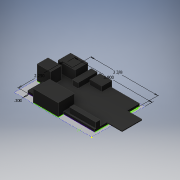
# Autodesk Inventor part: comp
Saved by Autodesk Inventor 2018 (Build 220112000, 112)
## iProperties
Created: 2018-03-12
Part Number: comp
Material: Generic
Document SubType Name: Modeling
Designer: Josh
Density: 1 g/cm^3
Appearance: Glossy - Black
Author: Josh
Autodesk Inventor part; units mm, degrees
ref_plane "YZ Plane" through (0, 0, 0) normal (1, 0, 0) x (0, 1, 0)
ref_plane "XZ Plane" through (0, 0, 0) normal (0, 1, 0) x (-1, 0, 0)
ref_plane "XY Plane" through (0, 0, 0) normal (0, 0, 1) x (1, 0, 0)
sketch "Sketch1" plane through (0, 0, 0) normal (0, 1, 0) x (-1, 0, 0)
  line L0 (0, 0) -> (99.06, 0) construction
  line L1 (99.06, 0) -> (99.06, -67.803) construction
  line L2 (99.06, -67.803) -> (0, -67.803) construction
  line L3 (0, -67.803) -> (0, 0) construction
  line L4 (3.6636, -7.62) -> (89.3886, -7.62)
  line L5 (89.3886, -7.62) -> (89.3886, -64.77)
  line L6 (89.3886, -64.77) -> (3.6636, -64.77)
  line L7 (3.6636, -64.77) -> (3.6636, -7.62)
  line L8 (79.4904, -27.0781) -> (96.8098, -27.0781)
  line L9 (96.8098, -27.0781) -> (96.8098, -40.9573)
  line L10 (96.8098, -40.9573) -> (79.4904, -40.9573)
  line L11 (79.4904, -40.9573) -> (79.4904, -27.0781)
  line L12 (90.7598, -47.719) -> (68.9327, -47.719)
  line L13 (68.9327, -47.719) -> (68.9327, -63.8522)
  line L14 (68.9327, -63.8522) -> (90.7598, -63.8522)
  line L15 (90.7598, -63.8522) -> (90.7598, -47.719)
  line L16 (55.7859, -66.2925) -> (40.4182, -66.2925)
  line L17 (40.4182, -66.2925) -> (40.4182, -53.4684)
  line L18 (40.4182, -53.4684) -> (55.7859, -53.4684)
  line L19 (55.7859, -53.4684) -> (55.7859, -66.2925)
  line L20 (9.1527, -52.5145) -> (2.1577, -52.5145)
  line L21 (2.1577, -52.5145) -> (2.1577, -61.4172)
  line L22 (2.1577, -61.4172) -> (9.1527, -61.4172)
  line L23 (9.1527, -61.4172) -> (9.1527, -52.5145)
  line L24 (37.3446, -14.572) -> (3.6636, -14.572)
  line L25 (3.6636, -14.572) -> (3.6636, -9.0608)
  line L26 (3.6636, -9.0608) -> (37.3446, -9.0608)
  line L27 (37.3446, -9.0608) -> (37.3446, -14.572)
  line L28 (43.4917, -21.567) -> (75.2871, -21.567)
  line L29 (75.2871, -21.567) -> (75.2871, -0.688)
  line L30 (75.2871, -0.688) -> (43.4917, -0.688)
  line L31 (43.4917, -0.688) -> (43.4917, -21.567)
  line L32 (66.6334, -41.9689) -> (59.3894, -41.9689)
  line L33 (59.3894, -41.9689) -> (59.3894, -66.2925)
  line L34 (59.3894, -66.2925) -> (66.6334, -66.2925)
  line L35 (66.6334, -66.2925) -> (66.6334, -41.9689)
  point P0 (15.875, 0)
  dimension "d6" = 99.06
  dimension "d18" = 85.725
  dimension "d19" = 57.15
  dimension "d20" = 7.62
  constraints: 64 end point, 16 parallel, 8 horizontal, 8 perpendicular, 2 point on line, 2 other
  measures "d6" distance of L1.end L2.end
  measures "d18" distance of L5.end L6.end
  measures "d19" distance of L4.end L5.end
  measures "d20" distance between parallel lines of L0 L4
extrude "Extrusion1" add sketch "Sketch1" along normal blind 3.175 contours L4 L31 L28 L29 L5 L8 L11 L10 L12 L13 L14 L6 L35 L32 L33 L19 L18 L17 L7 L22 L23 L20 L24 L27 L26 | L4 L29 L28 L31 | L26 L27 L24 L7 | L20 L23 L22 L7 | L5 L10 L11 L8 | L5 L14 L13 L12 | L17 L18 L19 L6 | L33 L32 L35 L6
extrude "Extrusion2" cut sketch "Sketch1" along normal blind 19.05 contours L8 L9 L10 L5 | L5 L10 L11 L8
extrude "Extrusion3" add sketch "Sketch1" along normal blind 19.05 contours L8 L9 L10 L5 | L5 L10 L11 L8
extrude "Extrusion4" cut sketch "Sketch1" along normal blind 15.875 contours L31 L30 L29 L4 | L4 L29 L28 L31
extrude "Extrusion5" add sketch "Sketch1" along normal blind 15.875 contours L31 L30 L29 L4 | L4 L29 L28 L31
extrude "Extrusion6" cut sketch "Sketch1" along normal blind 9.525 contours L17 L18 L19 L6 | L6 L19 L16 L17
extrude "Extrusion7" add sketch "Sketch1" along normal blind 9.525 contours L17 L18 L19 L6 | L6 L19 L16 L17
extrude "Extrusion8" cut sketch "Sketch1" along normal blind 9.525 contours L33 L32 L35 L6 | L6 L35 L34 L33
extrude "Extrusion9" add sketch "Sketch1" along normal blind 9.525 contours L33 L32 L35 L6 | L6 L35 L34 L33
extrude "Extrusion10" cut sketch "Sketch1" along normal blind 15.875 contours L12 L15 L14 L5 | L5 L14 L13 L12
extrude "Extrusion11" add sketch "Sketch1" along normal blind 15.875 contours L12 L15 L14 L5 | L5 L14 L13 L12
sketch "Sketch2" plane through (0, 0, 0) normal (0, -1, 0) x (1, 0, 0)
  point P0 (0, 0)
extrude "Extrusion12" cut sketch "Sketch1" along normal blind 10.16 contours L26 L27 L24 L7
extrude "Extrusion13" add sketch "Sketch1" along normal blind 10.16 contours L26 L27 L24 L7
sketch "Sketch3" plane through (0, 3.175, 0) normal (0, 1, 0) x (1, 0, 0)
  line L0 (-3.6636, 14.572) -> (-3.6636, 64.77) projected
  line L1 (-3.6636, 48.895) -> (15.3864, 48.895)
  line L2 (15.3864, 48.895) -> (15.3864, 23.495)
  line L3 (15.3864, 23.495) -> (-3.6636, 23.495)
  line L4 (-3.6636, 23.495) -> (-3.6636, 48.895)
  point P0 (0, 0)
  dimension "d49" = 15.875
  dimension "d50" = 19.05
  dimension "d51" = 25.4
  constraints: 8 end point, 2 parallel, 1 horizontal, 1 perpendicular, 1 point on line
  measures "d49" distance of L0.end L1.start
  measures "d50" distance of L2.end L3.end
  measures "d51" distance of L1.end L2.end
extrude "Extrusion14" add sketch "Sketch3" against normal blind 1.27
body "Solid1"
